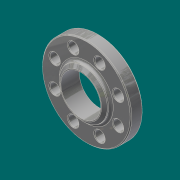
# Autodesk Inventor part: A1-19027-400-08 Alco flange - 2in CL300
Saved by Autodesk Inventor 2017.3 (Build 213257000, 257)
## iProperties
Created: 2019-06-24
Part Number: A1-19027-400-08 Alco flange - 2in CL300
Material: Steel, Mild
Document SubType Name: Modeling
Designer: Graeme_Van_Dongen
Density: 7.85 g/cm^3
Appearance: Steel
Mass: 2804.81 g
Surface Area: 607.208 cm^2
Volume: 357.3 cm^3
Description: 2" CLASS 300 RF ALCO FLANGE, A105N, Ø2.90" BORE, MATES TO B16.5 CLASS 300
Author: Graeme_Van_Dongen
Autodesk Inventor part; units mm, degrees
ref_plane "YZ Plane" through (0, 0, 0) normal (1, 0, 0) x (0, 1, 0)
ref_plane "XZ Plane" through (0, 0, 0) normal (0, 1, 0) x (-1, 0, 0)
ref_plane "XY Plane" through (0, 0, 0) normal (0, 0, 1) x (1, 0, 0)
sketch "Sketch1" plane through (0, 0, 0) normal (1, 0, 0) x (0, 1, 0)
  line L0 (0, 0) -> (0, 34.1313)
  line L1 (46.0375, 0) -> (36.83, 0)
  line L2 (36.83, 0) -> (36.83, 34.1313)
  line L3 (36.83, 34.1313) -> (38.4175, 34.1313)
  line L4 (38.4175, 34.1313) -> (44.45, 29.5023)
  line L5 (44.45, 29.5023) -> (44.8971, 27.6812)
  arc A0 (44.8971, 27.6812) -> (49.8306, 23.8125) centre (49.8306, 28.8925) ccw
  line L6 (49.8306, 23.8125) -> (82.55, 23.8125)
  line L7 (82.55, 23.8125) -> (82.55, 1.5875)
  line L8 (82.55, 1.5875) -> (46.0375, 1.5875)
  line L9 (46.0375, 1.5875) -> (46.0375, 0)
  point P0 (45.847, 23.8125)
  dimension "d0" = 34.1313
  dimension "d1" = 165.1
  dimension "d2" = 23.8125
  dimension "d3" = 92.075
  dimension "d4" = 1.5875
  dimension "d5" = 88.9
  dimension "d6" = 73.66
  dimension "d7" = 91.694
  dimension "d8" = 37.5
  dimension "d9" = 6.0325
  dimension "d10" = 5.08
  constraints: 20 end point, 5 perpendicular, 4 point on line, 2 point on circle, 2 tangent, 1 centre point, 1 horizontal, 1 parallel, 1 vertical
  measures "d0" distance of L0.start L0.end
  measures "d1" diameter of L7 L0
  measures "d2" distance between parallel lines of L6 L1
  measures "d3" diameter of L9 L0
  measures "d4" distance between parallel lines of L8 L1
  measures "d5" diameter of L4.end L0
  measures "d6" diameter of L2 L0
  measures "d7" diameter of point (45.847, 23.812) L0
  measures "d8" angle of L3 L4
  measures "d9" horizontal distance of L3.end L4.end
  measures "d10" radius of A0
revolve "Revolution1" add sketch "Sketch1" angle 360 about axis through (0, 0, 0) along (0, 0, 1)
sketch "Sketch2" plane through (0, 0, 23.8125) normal (0, 0, 1) x (1, 0, 0)
  line L0 (0, -115.57) -> (0, 115.57) construction
  line L1 (-24.3004, -58.6664) -> (24.3004, 58.6664) construction
  point P0 (0, 0)
  dimension "d12" = 127
  dimension "d13" = 22.5
  constraints: 2 end point, 1 coincident, 1 midpoint
  measures "d12" distance of L1.start L1.end
  measures "d13" angle of L0 L1
hole "Hole1" at (24.3004, 58.6664, 23.8125) direction (0, 0, -1) diameter 19.05 end through all
chamfer "Chamfer1" distance 1.1906 angle 45 2 edges at (24.3004, 68.1914, 23.8125) (24.3004, 68.1914, 1.5875)
pattern_circular "Circular Pattern1" count 8 over 360 about axis through (0, 0, -10) along (0, 0, 1) of "Hole1", "Chamfer1"
chamfer "Chamfer2" distance 1.5875 angle 45 2 edges at (0, -82.55, 23.8125) (0, -82.55, 1.5875)
equation "\"d0\" = Length"
equation "\"d1\" = OutsideDiameter"
equation "\"d2\" = Thickness"
equation "\"d3\" = RFDiameter"
equation "\"d4\" = RFThickness"
equation "\"d5\" = CasingDiameter"
equation "\"d6\" = Bore"
equation "\"d7\" = HubDiameter"
equation "\"d8\" = WeldBevelAngle"
equation "\"d9\" = WeldBevelSize"
equation "\"d10\" = HubRadius"
equation "\"d12\" = BCD"
equation "\"d14\" = HoleDiameter"
equation "\"d21\" = HoleChamfer"
equation "\"d27\" = RimChamfer"
equation "\"OutsideDiameter\" = 165.1"
equation "\"Thickness\" = 23.8125"
equation "\"Length\" = 34.13125"
equation "\"RFDiameter\" = 92.075"
equation "\"CasingDiameter\" = 88.9"
equation "\"Bore\" = 73.66"
equation "\"HoleDiameter\" = 19.05"
equation "\"BCD\" = 127"
equation "\"RFThickness\" = 1.5875"
equation "\"WeldBevelAngle\" = 37.5deg"
equation "\"HubDiameter\" = 91.694"
equation "\"HoleChamfer\" = 1.19063"
equation "\"RimChamfer\" = 1.5875"
equation "\"HubRadius\" = 5.08"
equation "\"WeldBevelSize\" = 6.0325"
body "Solid1"
